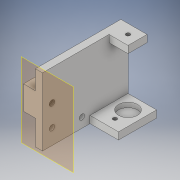
# Autodesk Inventor part: WheelIntake4.0Base
Saved by Autodesk Inventor 2017 SP1 (Build 210196100, 196)
## iProperties
Created: 2017-12-13
Part Number: WheelIntake4.0Base
Material: Generic
Document SubType Name: Modeling
Designer: User
Density: 1 g/cm^3
Appearance: Default
Author: User
Autodesk Inventor part; units mm, degrees
ref_plane "YZ Plane" through (0, 0, 0) normal (1, 0, 0) x (0, 1, 0)
ref_plane "XZ Plane" through (0, 0, 0) normal (0, 1, 0) x (-1, 0, 0)
ref_plane "XY Plane" through (0, 0, 0) normal (0, 0, 1) x (1, 0, 0)
sketch "Sketch1" plane through (0, 0, 0) normal (1, 0, 0) x (0, 1, 0)
  line L0 (0, 0) -> (45.2437, 0)
  line L1 (45.2437, 0) -> (45.2438, -57.15)
  line L2 (45.2438, -57.15) -> (0, -57.15)
  line L3 (0, -57.15) -> (0, 0)
  dimension "d0" = 45.2437
  dimension "d1" = 57.15
  constraints: 8 end point, 2 parallel, 1 horizontal, 1 perpendicular
  measures "d0" distance of L1.end L2.end
  measures "d1" distance of L0.end L1.end
extrude "Extrusion1" add sketch "Sketch1" along normal blind 4.7625
sketch "Sketch2" plane through (4.7625, 0, 0) normal (1, 0, 0) x (0, 0, -1)
  line L0 (0, 45.2437) -> (0, 0) projected
  line L1 (0, 0) -> (57.15, 0) projected
  line L2 (57.15, 0) -> (57.15, 45.2438) projected
  line L3 (57.15, 45.2438) -> (0, 45.2437) projected
  line L4 (0, 45.2437) -> (12.7, 45.2437)
  line L5 (12.7, 45.2437) -> (12.7, 40.4812)
  line L6 (12.7, 40.4812) -> (0, 40.4812)
  line L7 (0, 40.4812) -> (0, 45.2437)
  dimension "d4" = 12.7
  dimension "d5" = 4.7625
  constraints: 8 end point, 2 parallel, 1 horizontal, 1 perpendicular
  measures "d4" distance of L5.end L6.end
  measures "d5" distance of L4.end L5.end
extrude "Extrusion2" add sketch "Sketch2" along normal blind 12.7 contours L3 L5 L6 L0
sketch "Sketch3" plane through (4.7625, 0, 0) normal (1, 0, 0) x (0, 0, -1)
  line L0 (12.7, 40.4812) -> (0, 40.4812) projected
  line L1 (0, 40.4812) -> (0, 0) projected
  line L2 (0, 0) -> (57.15, 0) projected
  line L3 (57.15, 0) -> (57.15, 45.2438) projected
  line L4 (57.15, 45.2438) -> (12.7, 45.2437) projected
  line L5 (12.7, 45.2437) -> (12.7, 40.4812) projected
  line L6 (0, 0) -> (25.4, 0)
  line L7 (25.4, 0) -> (25.4, 4.7625)
  line L8 (25.4, 4.7625) -> (0, 4.7625)
  line L9 (0, 4.7625) -> (0, 0)
  dimension "d8" = 4.7625
  constraints: 8 end point, 2 parallel, 1 horizontal, 1 perpendicular
  measures "d8" distance of L7.end L6.end
extrude "Extrusion3" add sketch "Sketch3" along normal blind 19.05 contours L8 L7 L2 L1
sketch "Sketch4" plane through (0, 0, 0) normal (-1, 0, 0) x (0, 0, 1)
  line L0 (0, 0) -> (0, 45.2437) projected
  line L1 (0, 45.2437) -> (-57.15, 45.2438) projected
  line L2 (-57.15, 45.2438) -> (-57.15, 0) projected
  line L3 (-57.15, 0) -> (0, 0) projected
  line L4 (-57.15, 45.2438) -> (-12.7, 45.2437) projected
  line L5 (-57.15, 45.2438) -> (-44.45, 45.2438)
  line L6 (-57.15, 29.3688) -> (-57.15, 45.2438)
  line L7 (-57.15, 0) -> (-57.15, 45.2438) projected
  line L8 (-57.15, 32.5438) -> (-44.45, 32.5438)
  line L9 (-44.45, 32.5438) -> (-44.45, 16.6688)
  line L10 (-44.45, 16.6688) -> (-57.15, 16.6688)
  line L11 (-57.15, 16.6688) -> (-57.15, 32.5438)
  dimension "d48" = 15.875
  dimension "d49" = 12.7
  dimension "d50" = 12.7
  constraints: 12 end point, 2 horizontal, 2 parallel, 1 perpendicular, 1 point on line
  measures "d48" distance of L8.end L9.end
  measures "d49" distance between parallel lines of L1 L8
  measures "d50" distance of L8.start L8.end
extrude "Extrusion4" add sketch "Sketch4" along normal blind 7.9375 contours L2 L8 L9 L10
sketch "Sketch5" plane through (4.7625, 0, 0) normal (1, 0, 0) x (0, 0, -1)
  line L0 (25.4, 4.7625) -> (25.4, 0) projected
  line L1 (25.4, 0) -> (57.15, 0) projected
  line L2 (57.15, 0) -> (57.15, 45.2438) projected
  line L3 (57.15, 45.2438) -> (12.7, 45.2437) projected
  line L4 (12.7, 45.2437) -> (12.7, 40.4812) projected
  line L5 (12.7, 40.4812) -> (0, 40.4812) projected
  line L6 (0, 40.4812) -> (0, 4.7625) projected
  line L7 (0, 4.7625) -> (25.4, 4.7625) projected
  line L8 (0, 45.2437) -> (0, 40.4812) projected
  line L9 (0, 40.4812) -> (12.7, 40.4812) projected
  line L10 (12.7, 40.4812) -> (12.7, 45.2437) projected
  line L11 (12.7, 45.2437) -> (0, 45.2437) projected
  point P0 (0, 0)
  point P1 (50.8, 24.6063)
  dimension "d15" = 4.7625
  dimension "d16" = 20.6375
  dimension "d17" = 6.35
  measures "d15" distance of L3.end L4.end
  measures "d16" distance from line of L3 point (50.8, 24.606)
  measures "d17" distance from line of L2 point (50.8, 24.606)
hole "Hole1" at (4.7625, 24.6063, -50.8) direction (-1, 0, 0) diameter 3.683 depth 14.9352 tip angle 118 thread size "10-24 UNC" class "2B" standard "ANSI Unified Screw Threads"
sketch "Sketch6" plane through (4.7625, 4.7625, 0) normal (0, 1, 0) x (1, 0, 0)
  line L0 (0, 0) -> (0, 25.4) projected
  line L1 (0, 0) -> (19.05, 0) projected
  line L2 (19.05, 25.4) -> (19.05, 0) projected
  line L3 (0, 25.4) -> (19.05, 25.4) projected
  point P0 (-4.7625, 0)
  point P1 (9.525, 9.525)
  dimension "d25" = 9.525
  dimension "d26" = 9.525
  measures "d25" distance from line of L0 point (9.525, 9.525)
  measures "d26" distance from line of L1 point (9.525, 9.525)
hole "Hole2" at (14.2875, 4.7625, -9.525) direction (0, -1, 0) diameter 12.7 depth 3.175
sketch "Sketch10" plane through (0, 45.2438, 0) normal (0, 1, 0) x (1, 0, 0)
  line L0 (0, 0) -> (0, 57.15) projected
  line L1 (0, 0) -> (17.4625, 0) projected
  line L2 (17.4625, 12.7) -> (17.4625, 0) projected
  line L3 (4.7625, 12.7) -> (17.4625, 12.7) projected
  line L4 (4.7625, 57.15) -> (4.7625, 12.7) projected
  line L5 (0, 57.15) -> (4.7625, 57.15) projected
  point P0 (0, 0)
  point P1 (11.1125, 6.35)
hole "Hole3" at (11.1125, 45.2438, -6.35) direction (0, -1, 0) diameter 2.6416 depth 10.9728 tip angle 118 thread size "6-32 UNC" class "2B" standard "ANSI Unified Screw Threads"
sketch "Sketch11" plane through (0, 0, -57.15) normal (0, -1, 0) x (1, 0, 0)
  line L0 (0, 0) -> (0, 57.15) projected
  line L1 (0, 0) -> (4.7625, 0) projected
  line L2 (4.7625, 31.75) -> (4.7625, 0) projected
  line L3 (4.7625, 31.75) -> (23.8125, 31.75) projected
  line L4 (23.8125, 57.15) -> (23.8125, 31.75) projected
  line L5 (0, 57.15) -> (23.8125, 57.15) projected
  point P0 (15.0812, 38.1)
  dimension "d58" = 6.35
  measures "d58" distance from line of L3 point (15.081, 38.1)
hole "Hole4" at (15.0812, 0, -19.05) direction (0, 1, 0) diameter 2.6416 depth 10.9728 tip angle 118 thread size "6-32 UNC" class "2B" standard "ANSI Unified Screw Threads"
ref_plane "Work Plane1" through (-7.9375, 32.5438, -57.15) normal (0, 0, 1) x (0, -1, 0)
mirror "Mirror1" about plane through (-7.9375, 32.5438, -57.15) normal (0, 0, 1) remove original yes
sketch "Sketch12" plane through (4.7625, 0, -57.15) normal (1, 0, 0) x (0, 0, -1)
  circle A0 centre (6.35, 24.6062) radius 1.8415 projected
  line L0 (31.75, 4.7625) -> (31.75, 0) projected
  line L1 (57.15, 4.7625) -> (31.75, 4.7625) projected
  line L2 (57.15, 40.4812) -> (57.15, 4.7625) projected
  line L3 (44.45, 40.4812) -> (57.15, 40.4812) projected
  line L4 (44.45, 45.2437) -> (44.45, 40.4812) projected
  line L5 (0, 45.2437) -> (44.45, 45.2437) projected
  line L6 (0, 0) -> (0, 45.2437) projected
  line L7 (31.75, 0) -> (0, 0) projected
  point P0 (-57.15, 0)
  point P1 (6.35, 10.3124)
  point P2 (26.3525, 6.5024)
  dimension "d66" = 10.3124
  dimension "d67" = 6.35
  dimension "d68" = 6.5024
  dimension "d69" = 26.3525
  measures "d66" distance from line of L7 point (6.35, 10.312)
  measures "d67" distance from line of L6 point (6.35, 10.312)
  measures "d68" distance from line of L7 point (26.352, 6.502)
  measures "d69" distance from line of L6 point (26.352, 6.502)
hole "Hole5" at (4.7625, 10.3124, -63.5) at (4.7625, 6.5024, -83.5025) direction (-1, 0, 0) diameter 3.556 end through all
body "Solid1"
